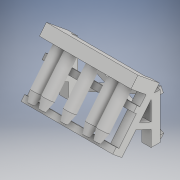
# Autodesk Inventor part: solar heater 2
Saved by Autodesk Inventor 2019 (Build 230136000, 136)
## iProperties
Created: 2019-06-15
Part Number: solar heater 2
Material: Generic
Document SubType Name: Modeling
Designer: Admin
Density: 1 g/cm^3
Appearance: Default
Author: Admin
Autodesk Inventor part; units mm, degrees
sketch "Sketch1" plane through (0, 0, 0) normal (0, 1, 0) x (-1, 0, 0)
  line L0 (0, 0) -> (250, 0)
  line L1 (250, 0) -> (250, -50)
  line L2 (250, -50) -> (0, -50)
  line L3 (0, -50) -> (0, 0)
  line L4 (0, -500) -> (250, -500)
  line L5 (250, -500) -> (250, -450)
  line L6 (250, -450) -> (0, -450)
  line L7 (0, -450) -> (0, -500)
  dimension "d0" = 250
  dimension "d1" = 50
  dimension "d2" = 250
  dimension "d3" = 50
  constraints: 16 end point, 4 parallel, 2 horizontal, 2 perpendicular
  measures "d0" distance of L1.end L2.end
  measures "d1" distance of L0.end L1.end
  measures "d2" distance of L6.end L5.end
  measures "d3" distance of L5.end L4.end
extrude "Extrusion1" add sketch "Sketch1" along normal blind 50
sketch "Sketch2" plane through (0, 50, 0) normal (0, 1, 0) x (1, 0, 0)
  line L0 (-250, 15.445209) -> (-27.801378, 500)
  line L1 (-27.801378, 500) -> (-0.163961, 487.326519)
  line L2 (-0.163961, 487.326519) -> (-222.362583, 2.771728)
  line L3 (-222.362583, 2.771728) -> (-250, 15.445209)
  line L4 (-250, 477.771798) -> (-33.979462, 0)
  line L5 (-33.979462, 0) -> (-2.366854, 14.293377)
  line L6 (-2.366854, 14.293377) -> (-218.387392, 492.065175)
  line L7 (-218.387392, 492.065175) -> (-250, 477.771798)
  constraints: 16 end point, 4 parallel, 2 perpendicular
extrude "Extrusion2" add sketch "Sketch2" along normal blind 20
sketch "Sketch3" plane through (-250, 0, 0) normal (0, 0, 1) x (1, 0, 0)
  line L0 (-32.538476, 45.433012) -> (217.853804, -159.054018)
  line L1 (217.853804, -159.054018) -> (189.247428, -194.082234)
  line L2 (189.247428, -194.082234) -> (-61.144852, 10.404797)
  line L3 (-61.144852, 10.404797) -> (-32.538476, 45.433012)
  point P0 (250, 0)
  constraints: 8 end point, 2 parallel, 1 perpendicular
extrude "Extrusion3" add sketch "Sketch3" against normal blind 500
sketch "Sketch4" plane through (0, 0, 0) normal (0, 0, 1) x (1, 0, 0)
  line L0 (-169.808572, -105.019833) -> (-100.396682, 45.41755)
  line L1 (-100.396682, 45.41755) -> (-71.745385, 32.197826)
  line L2 (-71.745385, 32.197826) -> (-141.157275, -118.239557)
  line L3 (-141.157275, -118.239557) -> (-169.808572, -105.019833)
  point P0 (0, 0)
  constraints: 8 end point, 2 parallel, 1 perpendicular
extrude "Extrusion4" add sketch "Sketch4" against normal blind 50
sketch "Sketch5" plane through (0, 0, -500) normal (0, 0, -1) x (-1, 0, 0)
  line L0 (164.991709, -94.580176) -> (105.992311, 33.290063)
  line L1 (105.992311, 33.290063) -> (77.190635, 20.000954)
  line L2 (77.190635, 20.000954) -> (136.190033, -107.869285)
  line L3 (136.190033, -107.869285) -> (164.991709, -94.580176)
  line L4 (150.240723, -62.610154) -> (121.352364, 0)
  point P0 (0, 0)
  constraints: 8 end point, 2 parallel, 1 collinear, 1 perpendicular
extrude "Extrusion5" add sketch "Sketch5" against normal blind 50
sketch "Sketch7" plane through (-311.144852, 10.404797, -500) normal (-0.6325346, -0.7745321, 0) x (0.7745321, -0.6325346, 0)
  line L0 (500, 54.190895) -> (0, 54.190895)
  line L1 (0, 54.190895) -> (0, 454.190895)
  line L2 (0, 454.190895) -> (500, 454.190895)
  line L3 (500, 454.190895) -> (500, 54.190895)
  point P0 (247.573076, 500)
  dimension "d14" = 400
  constraints: 8 end point, 2 parallel, 1 horizontal, 1 perpendicular
  measures "d14" distance of L0.end L1.end
extrude "Extrusion6" cut sketch "Sketch7" against normal blind 50
sketch "Sketch8" plane through (-311.144852, 10.404797, -500) normal (-0.6325346, -0.7745321, 0) x (0.7745321, -0.6325346, 0)
  line L0 (112.704347, 500) -> (142.704347, 500)
  line L1 (142.704347, 500) -> (142.704347, 0)
  line L2 (142.704347, 0) -> (112.704347, 0)
  line L3 (112.704347, 0) -> (112.704347, 500)
  point P0 (247.573076, 500)
  dimension "d17" = 30
  constraints: 8 end point, 2 parallel, 1 horizontal, 1 perpendicular
  measures "d17" distance of L1.end L2.end
extrude "Extrusion7" add sketch "Sketch8" along normal blind 20
sketch "Sketch9" plane through (-60.752572, -194.082234, -500) normal (-0.6325346, -0.7745321, 0) x (0.7745321, -0.6325346, 0)
  line L0 (0, 500) -> (-30, 500)
  line L1 (-30, 500) -> (-30, 0)
  line L2 (-30, 0) -> (0, 0)
  line L3 (0, 0) -> (0, 500)
  point P0 (-75.708904, 500)
  dimension "d20" = 30
  constraints: 8 end point, 2 parallel, 1 horizontal, 1 perpendicular
  measures "d20" distance of L2.end L1.end
extrude "Extrusion8" add sketch "Sketch9" along normal blind 20
sketch "Sketch10" plane through (0, 0, -500) normal (0, 0, -1) x (-1, 0, 0)
  line L0 (311.144852, 10.404797) -> (343.264293, -28.925132)
  line L1 (343.264293, -28.925132) -> (296.792366, -66.877206)
  line L2 (296.792366, -66.877206) -> (264.672924, -27.547278)
  line L3 (264.672924, -27.547278) -> (311.144852, 10.404797)
  point P0 (0, 0)
  dimension "d23" = 60
  constraints: 8 end point, 2 parallel, 1 perpendicular
  measures "d23" distance of L0.end L1.end
extrude "Extrusion9" add sketch "Sketch10" against normal blind 500
sketch "Sketch11" plane through (-296.792366, -66.877206, 0) normal (0.7745321, -0.6325346, 0) x (0, 0, -1)
  circle A0 centre (250, 0) radius 28.868524
  point P0 (0, 239.529978)
  constraints: 1 centre point
extrude "Extrusion10" add sketch "Sketch11" along normal blind 200
sketch "Sketch12" plane through (0, 0, -500) normal (0, 0, -1) x (-1, 0, 0)
  line L0 (264.672924, -27.547278) -> (331.574676, -109.467789)
  line L1 (331.574676, -109.467789) -> (378.046603, -71.515715)
  line L2 (378.046603, -71.515715) -> (311.144852, 10.404797)
  line L3 (311.144852, 10.404797) -> (264.672924, -27.547278)
  point P0 (0, 0)
  dimension "d28" = 60
  constraints: 8 end point, 2 parallel, 1 perpendicular
  measures "d28" distance of L1.end L0.end
extrude "Extrusion11" add sketch "Sketch12" against normal blind 500
ref_plane "Work Plane1" through (-103.159335, -225.01085, -250) normal (0.7745321, -0.6325346, 0) x (0, 0, -1)
sketch "Sketch14" plane through (-103.159335, -225.01085, -250) normal (0.7745321, -0.6325346, 0) x (0, 0, -1)
  circle A0 centre (0, 0) radius 15
  point P0 (-250, 239.529978)
  dimension "d32" = 30
  constraints: 1 centre point
  measures "d32" diameter of A0
loft "Loft1" add profiles "Sketch14" section 1 edges at (-141.885941, -193.384121, -221.131476)
ref_plane "Work Plane2" through (0, 0, -190) normal (0, 0, 1) x (1, 0, 0)
mirror "Mirror1" about plane through (0, 0, -190) normal (0, 0, 1) of "Extrusion10"
mirror "Mirror2" about plane through (0, 0, -190) normal (0, 0, 1) of "Loft1"
ref_plane "Work Plane3" through (0, 0, -100) normal (0, 0, 1) x (1, 0, 0)
mirror "Mirror5" about plane through (0, 0, -100) normal (0, 0, 1) of "Extrusion10", "Mirror1"
mirror "Mirror6" about plane through (0, 0, -100) normal (0, 0, 1) of "Loft1", "Mirror2"
sketch "Sketch17" plane through (-103.159335, -225.01085, 50) normal (0.7745321, -0.6325346, 0) x (0, 0, -1)
  circle A0 centre (0, 0) radius 15
  circle A1 centre (0, 0) radius 43.471227
  point P0 (50, 239.529978)
  constraints: 1 centre point, 1 coincident
extrude "Extrusion13" cut sketch "Sketch17" against normal blind 500
sketch "Sketch18" plane through (-103.159335, -225.01085, 50) normal (0.7745321, -0.6325346, 0) x (0, 0, -1)
  circle A0 centre (0, 0) radius 35.71998
  point P0 (50, 239.529978)
  constraints: 1 centre point
extrude "Extrusion14" cut sketch "Sketch18" against normal blind 500
ref_plane "Work Plane5" through (0, 0, -310) normal (0, 0, -1) x (-1, 0, 0)
mirror "Mirror7" about plane through (0, 0, -310) normal (0, 0, -1) of "Extrusion10"
mirror "Mirror8" about plane through (0, 0, -310) normal (0, 0, -1) of "Loft1"
ref_plane "Work Plane6" through (0, 0, -400) normal (0, 0, -1) x (-1, 0, 0)
mirror "Mirror9" about plane through (0, 0, -400) normal (0, 0, -1) of "Extrusion10", "Mirror7"
mirror "Mirror10" about plane through (0, 0, -400) normal (0, 0, -1) of "Loft1", "Mirror8"
sketch "Sketch19" plane through (-103.159335, -225.01085, -550) normal (0.7745321, -0.6325346, 0) x (0, 0, -1)
  circle A0 centre (0, 0) radius 44.246955
  point P0 (-550, 239.529978)
  constraints: 1 centre point, 1 coincident
extrude "Extrusion15" cut sketch "Sketch19" against normal blind 500
body "Solid1"
